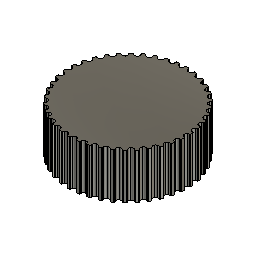
gear_42z (Autodesk Fusion 360 design; units mm, degrees)
Autodesk Fusion 360 part; units mm, degrees
sketch "Sketch1" plane through (0, 0, 0) normal (0, 0, 1) x (1, 0, 0) in component "gt2 pulley"
  circle A0 centre (0, 0) radius 13.369 construction
  circle A1 centre (0, 0) radius 12.365 construction
  line L0 (0, 0) -> (0, 13.369) construction
  line L1 (0, 0) -> (0.9991, 13.3316) construction
  line L2 (0, 0) -> (1.4082, 13.2946) construction
  circle A2 centre (0, 0) radius 13.115 construction
  arc A3 (0.3838, 12.9732) -> (0.4468, 12.6866) centre (1.3815, 13.0421) ccw
  circle A4 centre (0, 0) radius 12.965 construction
  arc A5 (0.2368, 13.1129) -> (0, 13.115) centre (0, 0) ccw
  arc A6 (0.3838, 12.9732) -> (0.2368, 13.1129) centre (0.2342, 12.9629) ccw
  arc A7 (0.4468, 12.6866) -> (0.924, 12.3304) centre (0.9655, 12.8839) ccw
  arc A8 (0, 13.115) -> (-0.2368, 13.1129) centre (0, 0) ccw
  arc A9 (-0.2368, 13.1129) -> (-0.3838, 12.9732) centre (-0.2342, 12.9629) ccw
  arc A10 (-0.4468, 12.6866) -> (-0.3838, 12.9732) centre (-1.3815, 13.0421) ccw
  arc A11 (-0.924, 12.3304) -> (-0.4468, 12.6866) centre (-0.9655, 12.8839) ccw
  arc A12 (0.924, 12.3304) -> (-0.924, 12.3304) centre (0, 0) ccw
  point P0 (1.3815, 13.0421)
  point P1 (0, 13.115)
  dimension "d18" = 26.738
  dimension "d19" = 4.286
  dimension "d22" = 1.004
  dimension "d24" = 0.75
  dimension "d26" = 1
  dimension "d27" = 0.15
  dimension "d28" = 0.15
  dimension "d47" = 0.555
  dimension "d52" = 3.812
  constraint coincident A0.centre A1.centre
  constraint coincident A0 L0.end
  constraint vertical L0
  constraint coincident A0 L1.end
  constraint coincident A0 L2.end
  constraint concentric A1 A2
  constraint coincident A1 A7.end
  constraint coincident L1 A7.end
  constraint coincident A2 P0
  constraint coincident L2 P0
  constraint coincident P0 A3.centre
  constraint coincident A2 P1
  constraint coincident L0 P1
  constraint concentric A2 A4
  constraint coincident P1 A5.end
  constraint coincident A4 A6.centre
  constraint coincident A3.start A6.start
  constraint tangent A3 A6
  constraint tangent A3 A7
  constraint symmetric L0 A7.end A11.start
  constraint symmetric L0 A3.start A9.end
  constraint symmetric L0 A3.end A10.start
  constraint symmetric L0 A3 A10
  constraint symmetric L0 A5.start A8.end
  constraint symmetric L0 P1 A5.end
  constraint symmetric L0 A5 A8
  constraint symmetric L0 A6 A9
  constraint symmetric L0 A7 A11
  constraint coincident A1 A11.start
  constraint tangent A1 A7
  constraint coincident L1 A7.centre
  measures "d18" diameter of A0
  measures "d19" angle of L0 L1
  measures "d22" distance of A0 A1
  measures "d24" distance of A1 A2
  measures "d26" radius of A3
  measures "d27" distance of A2 A4
  measures "d28" radius of A6
  measures "d47" radius of A7
extrude "Extrude1" add sketch "Sketch1" along normal blind 10 makes body 1
pattern_circular "C-Pattern1" count 42 over 360 about axis through (0, 0, 1.75) along (0, 0, 1) of bodies 1 makes body 2 at (-1.1289, 12.3134, 3.3333) makes body 3 at (-3.7427, 11.785, 6.6667) makes body 4 at (-5.4574, 11.0955, 6.6667) makes body 5 at (-7.0501, 10.1582, 6.6667) makes body 6 at (-8.4854, 8.994, 6.6667) makes body 7 at (-9.7311, 7.6288, 6.6667) makes body 8 at (-11.0498, 5.5494, 6.6667) makes body 9 at (-11.7535, 3.8405, 6.6667) makes body 10 at (-12.0775, 2.6512, 6.6667) makes body 11 at (-12.2559, 1.6394, 3.3333) makes body 12 at (-12.3633, -0.2055, 3.3333) makes body 13 at (-12.0317, -2.8516, 6.6667) makes body 14 at (-11.2281, -5.1791, 6.6667) makes body 15 at (-10.6567, -6.2713, 6.6667) makes body 16 at (-10.0993, -7.1343, 3.3333) makes body 17 at (-8.3347, -9.1338, 6.6667) makes body 18 at (-6.8803, -10.274, 6.6667) makes body 19 at (-5.2722, -11.1847, 6.6667) makes body 20 at (-3.5463, -11.8456, 6.6667) makes body 21 at (-1.1289, -12.3134, 6.6667) makes body 22 at (0.1028, -12.3646, 6.6667) makes body 23 at (1.1289, -12.3134, 3.3333) makes body 24 at (3.7427, -11.785, 6.6667) makes body 25 at (4.7081, -11.4336, 3.3333) makes body 26 at (7.0501, -10.1582, 6.6667) makes body 27 at (7.8691, -9.5379, 3.3333) makes body 28 at (10.0993, -7.1343, 6.6667) makes body 29 at (10.3308, -6.7947, 3.3333) makes body 30 at (11.2281, -5.1791, 3.3333) makes body 31 at (11.8746, -3.4478, 3.3333) makes body 32 at (12.3633, -0.2055, 6.6667) makes body 33 at (12.3633, 0.2055, 3.3333) makes body 34 at (11.9303, 3.2499, 6.6667) makes body 35 at (11.7535, 3.8405, 3.3333) makes body 36 at (10.6567, 6.2713, 6.6667) makes body 37 at (9.6029, 7.7895, 6.6667) makes body 38 at (8.9232, 8.5598, 3.3333) makes body 39 at (6.3596, 10.6042, 6.6667) makes body 40 at (5.2722, 11.1847, 6.6667) makes body 41 at (4.3255, 11.5838, 3.3333) makes body 42 at (1.7412, 12.2418, 6.6667)
sketch "Sketch2" plane through (0, 0, 10) normal (0, 0, 1) x (-1, 0, 0)
  arc A0 (-7.6252, -10.5028) -> (-7.5824, -10.701) centre (-7.4958, -10.5785) ccw
  arc A1 (-7.5824, -10.701) -> (-7.1911, -10.9678) centre (0, 0) ccw
  arc A2 (-7.1911, -10.9678) -> (-6.9909, -10.9352) centre (-7.1088, -10.8424) ccw
  arc A3 (-6.7775, -10.7338) -> (-6.9909, -10.9352) centre (-6.2054, -11.5541) ccw
  arc A4 (-6.1825, -10.7084) -> (-6.7775, -10.7338) centre (-6.46, -11.1891) ccw
  arc A5 (-7.7095, -9.6674) -> (-6.1825, -10.7084) centre (0, 0) ccw
  arc A6 (-7.5158, -10.2305) -> (-7.7095, -9.6674) centre (-8.0555, -10.1013) ccw
  arc A7 (-7.6252, -10.5028) -> (-7.5158, -10.2305) centre (-8.4883, -9.9976) ccw
  circle A8 centre (0, 0) radius 12.365
  constraint coincident A1.centre A5.centre
extrude "Extrude2" add sketch "Sketch2" against normal blind 10 contours A5 A8 bodies 1 2 3 4 5 6 7 8 9 10 11 12 13 14 15 16 17 18 19 20 21 22 23 24 25 26 27 28 29 30 31 32 33 34 35 36 37 38 39 40 41 42
extrude "Extrude4" [suppressed] in component "gt2 pulley"
pattern_circular "C-Pattern7" [suppressed] in component "gt2 pulley"
extrude "Extrude3" [suppressed] in component "gt2 pulley"
pattern_circular "C-Pattern6" [suppressed] in component "gt2 pulley"
extrude "Extrude2'" [suppressed] in component "gt2 pulley"
pattern_circular "C-Pattern5" [suppressed] in component "gt2 pulley"
extrude "Extrude1'" [suppressed] in component "gt2 pulley"
pattern_circular "C-Pattern4" [suppressed] in component "gt2 pulley"
pattern_circular "C-Pattern3" [suppressed] in component "gt2 pulley"
pattern_circular "C-Pattern2" [suppressed] in component "gt2 pulley"
pattern_circular "C-Pattern1'" [suppressed] in component "gt2 pulley"
copy_body "Body->Comp1" [suppressed] in component "Component"
copy_body "Body->Comp2" [suppressed] in component "Component'"
copy_body "Body->Comp3" [suppressed] in component "Component''"
copy_body "Body->Comp4" [suppressed] in component "Component'''"
copy_body "Body->Comp5" [suppressed] in component "Component''''"
copy_body "Body->Comp6" [suppressed] in component "Component'''''"
copy_body "Body->Comp7" [suppressed] in component "Component''''''"
copy_body "Body->Comp8" [suppressed] in component "Component'''''''"
copy_body "Body->Comp9" [suppressed] in component "Component''''''''"
copy_body "Body->Comp10" [suppressed] in component "Component'''''''''"
copy_body "Body->Comp11" [suppressed] in component "Component''''''''''"
copy_body "Body->Comp12" [suppressed] in component "Component'''''''''''"
copy_body "Body->Comp13" [suppressed] in component "Component''''''''''''"
copy_body "Body->Comp14" [suppressed] in component "Component'''''''''''''"
copy_body "Body->Comp15" [suppressed] in component "Component''''''''''''''"
copy_body "Body->Comp16" [suppressed] in component "Component'''''''''''''''"
copy_body "Body->Comp17" [suppressed] in component "Component''''''''''''''''"
copy_body "Body->Comp18" [suppressed] in component "Component'''''''''''''''''"
copy_body "Body->Comp19" [suppressed] in component "Component''''''''''''''''''"
copy_body "Body->Comp20" [suppressed] in component "Component'''''''''''''''''''"
component "gt2 pulley" placed x (1, 0, 0) y (0, 1, 0) z (0, 0, 1) at (0, 0, 0)
equation "NumTeeth = 42" comment "min 20"
equation "ToothPitch = 2 mm"
equation "PullyDia = NumTeeth * ToothPitch / PI"
equation "ToothAng = ( ( 360 / NumTeeth ) * 1 deg )"
equation "TransOffsetAngle = ToothAng * 0.2"
equation "Sholulder_Radius = 0.15 mm"
equation "Root_Radius = 0.555 mm"
equation "TransRadius = 1 mm"
equation "ToolHeight = 0.75 mm"
equation "PLD = 0.254 mm"
equation "d18 = PullyDia"
equation "d19 = ToothAng / 2"
equation "d22 = PLD + ToolHeight"
equation "d24 = ToolHeight"
equation "d26 = TransRadius"
equation "d27 = Sholulder_Radius"
equation "d31 = NumTeeth"
equation "d33 = NumTeeth"
equation "d35 = NumTeeth"
equation "d37 = NumTeeth"
equation "d41 = NumTeeth"
equation "d45 = NumTeeth"
equation "d47 = Root_Radius"
equation "d50 = NumTeeth"
